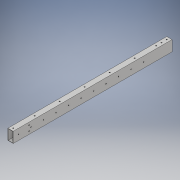
# Autodesk Inventor part: 1x2 30in
Saved by Autodesk Inventor 2018 (Build 220112000, 112)
## iProperties
Created: 2019-01-11
Part Number: 1x2 30in
Material: Generic
Document SubType Name: Modeling
Designer: s-2512711
Density: 1 g/cm^3
Appearance: Default
Author: s-2512711
Autodesk Inventor part; units mm, degrees
ref_plane "YZ Plane" through (0, 0, 0) normal (1, 0, 0) x (0, 1, 0)
ref_plane "XZ Plane" through (0, 0, 0) normal (0, 1, 0) x (-1, 0, 0)
ref_plane "XY Plane" through (0, 0, 0) normal (0, 0, 1) x (1, 0, 0)
sketch "Sketch1" plane through (0, 0, 0) normal (0, 0, 1) x (1, 0, 0)
  line L0 (0, 0) -> (25.4, 0)
  line L1 (25.4, 0) -> (25.4, 50.8)
  line L2 (25.4, 50.8) -> (0, 50.8)
  line L3 (0, 50.8) -> (0, 0)
  line L4 (23.8125, 49.2125) -> (23.8125, 1.5875)
  line L5 (23.8125, 1.5875) -> (1.5875, 1.5875)
  line L6 (1.5875, 1.5875) -> (1.5875, 49.2125)
  line L7 (1.5875, 49.2125) -> (23.8125, 49.2125)
  dimension "d0" = 25.4
  dimension "d1" = 50.8
  dimension "d2" = 1.5875
  constraints: 16 end point, 4 parallel, 2 perpendicular, 1 horizontal, 3 other
  measures "d0" distance of L2.end L1.end
  measures "d1" distance of L1.end L0.end
  measures "d2" distance between parallel lines of L1 L4
extrude "Extrusion1" add sketch "Sketch1" along normal blind 762
sketch "Sketch2" plane through (0, 0, 0) normal (0, -1, 0) x (1, 0, 0)
  line L0 (1.5875, 762) -> (23.8125, 762) construction
  line L1 (12.7, 762) -> (12.7, 646.6078) construction
  line L2 (12.7, 646.6078) -> (12.7, 526.6182) construction
  line L3 (12.7, 526.6182) -> (12.7, 406.6286) construction
  line L4 (12.7, 406.6286) -> (12.7, 286.639) construction
  line L5 (12.7, 286.639) -> (12.7, 166.6494) construction
  line L6 (23.8125, 0) -> (1.5875, 0) construction
  line L7 (12.7, 0) -> (12.7, 12.7) construction
  line L8 (12.7, 12.7) -> (12.7, 38.1) construction
  line L9 (12.7, 38.1) -> (12.7, 63.5) construction
  line L10 (12.7, 63.5) -> (12.7, 88.9) construction
  circle A0 centre (12.7, 12.7) radius 2.5797
  circle A1 centre (12.7, 38.1) radius 2.5797
  circle A2 centre (12.7, 63.5) radius 2.5797
  circle A3 centre (12.7, 166.6494) radius 2.5797
  circle A4 centre (12.7, 286.639) radius 2.5797
  circle A5 centre (12.7, 406.6286) radius 2.5797
  circle A6 centre (12.7, 526.6182) radius 2.5797
  circle A7 centre (12.7, 646.6078) radius 2.5797
  point P0 (0, 0)
  dimension "d5" = 115.3922
  dimension "d6" = 119.9896
  dimension "d7" = 119.9896
  dimension "d8" = 119.9896
  dimension "d9" = 119.9896
  dimension "d10" = 12.7
  dimension "d11" = 25.4
  dimension "d12" = 25.4
  dimension "d13" = 25.4
  dimension "d14" = 5.1594
  dimension "d15" = 5.1594
  dimension "d16" = 5.1594
  dimension "d18" = 5.1594
  dimension "d19" = 5.1594
  dimension "d20" = 5.1594
  dimension "d21" = 5.1594
  dimension "d22" = 5.1594
  constraints: 18 end point, 8 centre point, 7 point on line, 2 midpoint, 2 vertical, 1 coincident
  measures "d5" distance of L1.start L1.end
  measures "d6" distance of L1.end L2.end
  measures "d7" distance of L2.end L3.end
  measures "d8" distance of L3.end L4.end
  measures "d9" distance of L4.end L5.end
  measures "d10" distance of L7.start L7.end
  measures "d11" distance of L7.end L8.end
  measures "d12" distance of L8.end L9.end
  measures "d13" distance of L9.end L10.end
  measures "d14" diameter of A0
  measures "d15" diameter of A1
  measures "d16" diameter of A2
  measures "d18" diameter of A3
  measures "d19" diameter of A4
  measures "d20" diameter of A5
  measures "d21" diameter of A6
  measures "d22" diameter of A7
extrude "Extrusion3" cut sketch "Sketch2" against normal blind 134.9375
sketch "Sketch3" plane through (0, 50.8, 0) normal (0, 1, 0) x (1, 0, 0)
  line L0 (0, -762) -> (25.4, -762) construction
  line L1 (12.7, -762) -> (12.7, -749.3) construction
  circle A0 centre (12.7, -749.3) radius 2.5797
  point P0 (0, 0)
  dimension "d27" = 12.7
  dimension "d28" = 5.1594
  constraints: 2 end point, 1 centre point, 1 coincident, 1 midpoint, 1 vertical
  measures "d27" distance of L1.start L1.end
  measures "d28" diameter of A0
extrude "Extrusion4" cut sketch "Sketch3" against normal blind 525.4625
sketch "Sketch4" plane through (25.4, 0, 0) normal (1, 0, 0) x (0, 0, -1)
  line L0 (-762, 0) -> (-762, 50.8) construction
  line L1 (-762, 0) -> (-762, 12.7) construction
  line L2 (-762, 12.7) -> (-762, 38.1) construction
  line L3 (-762, 38.1) -> (-685.8, 38.1) construction
  line L4 (-762, 12.7) -> (-685.8, 12.7) construction
  circle A0 centre (-685.8, 38.1) radius 2.5797
  circle A1 centre (-685.8, 12.7) radius 2.5797
  point P0 (0, 0)
  dimension "d31" = 12.7
  dimension "d32" = 25.4
  dimension "d33" = 76.2
  dimension "d34" = 5.1594
  dimension "d37" = 76.2
  constraints: 8 end point, 2 centre point, 2 coincident, 2 point on line, 1 horizontal, 1 perpendicular
  measures "d31" distance of L0.start L1.end
  measures "d32" distance of L1.end L2.end
  measures "d33" distance of L2.end L3.end
  measures "d34" diameter of A0
  measures "d37" distance of L1.end L4.end
extrude "Extrusion5" cut sketch "Sketch4" against normal blind 25.4
sketch "Sketch5" plane through (25.4, 0, 0) normal (1, 0, 0) x (0, 0, -1)
  line L0 (0, 1.5875) -> (0, 49.2125) projected
  line L1 (0, 25.4) -> (-136.6, 25.4) construction
  line L2 (-136.6, 25.4) -> (-196.6, 25.4) construction
  line L3 (-196.6, 25.4) -> (-256.6, 25.4) construction
  line L4 (-256.6, 25.4) -> (-316.6, 25.4) construction
  line L5 (-316.6, 25.4) -> (-376.6, 25.4) construction
  line L6 (-376.6, 25.4) -> (-436.6, 25.4) construction
  line L7 (-436.6, 25.4) -> (-496.6, 25.4) construction
  line L8 (-496.6, 25.4) -> (-556.6, 25.4) construction
  line L9 (-556.6, 25.4) -> (-616.6, 25.4) construction
  line L10 (-616.6, 25.4) -> (-676.6, 25.4) construction
  line L11 (-676.6, 25.4) -> (-736.6, 25.4) construction
  line L12 (-736.6, 25.4) -> (-796.6, 25.4) construction
  circle A0 centre (-136.6, 25.4) radius 2.25
  circle A1 centre (-196.6, 25.4) radius 2.25
  circle A2 centre (-256.6, 25.4) radius 2.25
  circle A3 centre (-316.6, 25.4) radius 2.25
  circle A4 centre (-376.6, 25.4) radius 2.25
  circle A5 centre (-436.6, 25.4) radius 2.25
  circle A6 centre (-496.6, 25.4) radius 2.25
  circle A7 centre (-556.6, 25.4) radius 2.25
  circle A8 centre (-616.6, 25.4) radius 2.25
  circle A9 centre (-676.6, 25.4) radius 2.25
  circle A10 centre (-736.6, 25.4) radius 2.25
  point P0 (0, 0)
  dimension "d38" = 136.6
  dimension "d39" = 60
  dimension "d40" = 60
  dimension "d41" = 60
  dimension "d42" = 60
  dimension "d43" = 60
  dimension "d44" = 60
  dimension "d45" = 60
  dimension "d46" = 60
  dimension "d47" = 60
  dimension "d48" = 60
  dimension "d49" = 60
  dimension "d50" = 4.5
  constraints: 24 end point, 11 centre point, 11 coincident, 10 point on line, 2 horizontal, 1 midpoint
  measures "d38" distance of L1.start L1.end
  measures "d39" distance of L1.end L2.end
  measures "d40" distance of L2.end L3.end
  measures "d41" distance of L3.end L4.end
  measures "d42" distance of L4.end L5.end
  measures "d43" distance of L5.end L6.end
  measures "d44" distance of L6.end L7.end
  measures "d45" distance of L7.end L8.end
  measures "d46" distance of L8.end L9.end
  measures "d47" distance of L9.end L10.end
  measures "d48" distance of L10.end L11.end
  measures "d49" distance of L11.end L12.end
  measures "d50" diameter of A0
extrude "Extrusion6" cut sketch "Sketch5" against normal blind 25.4
body "Solid1"
